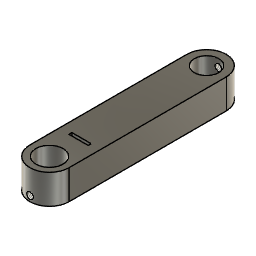
Stirrer Attachment v3 (Autodesk Fusion 360 design; units mm, degrees)
Autodesk Fusion 360 part; units mm, degrees
note: some values were not read from the file. Set by a fixed rule: which face or edge a step refers to.
sketch "Sketch1" plane through (0, 0, 0) normal (0, 0, 1) x (1, 0, 0)
  line L0 (10, -50) -> (-10, -50)
  line L1 (-10, -50) -> (-10, 50)
  line L2 (-10, 50) -> (10, 50)
  line L3 (10, 50) -> (10, -50)
  line L4 (10, -50) -> (-10, 50) construction
  line L5 (-10, -50) -> (10, 50) construction
  circle A0 centre (0, -40) radius 10
  circle A1 centre (0, 40) radius 10
  circle A2 centre (0, -40) radius 6.9
  line L6 (-2.5, -33.1) -> (2.5, -33.1)
  line L7 (0, -33.1) -> (0, -37.8)
  circle A3 centre (0, 40) radius 6.2
  line L8 (-4.7612, -23.8062) -> (5.065, -23.8062)
  line L9 (5.065, -23.8062) -> (5.065, -25.3251)
  line L10 (5.065, -25.3251) -> (-4.7612, -25.3251)
  line L11 (-4.7612, -25.3251) -> (-4.7612, -23.8062)
  dimension "d1" = 100
  dimension "d2" = 20
  dimension "d3" = 13.8
  dimension "d13" = 12.4
  constraint perpendicular L0 L1
  constraint parallel L0 L2
  constraint parallel L1 L3
  constraint horizontal L0
  constraint coincident L4 origin
  constraint coincident L5 origin
  constraint tangent L0 A0
  constraint tangent L1 A0
  constraint tangent L3 A0
  constraint tangent L2 A1
  constraint tangent L1 A1
  constraint tangent L3 A1
  constraint concentric A0 A2
  constraint horizontal L6
  constraint tangent A2 L6
  constraint midpoint L6 L7.start
  constraint perpendicular L6 L7
  constraint concentric A1 A3
  constraint horizontal L8
  constraint vertical L9
  constraint horizontal L10
  constraint vertical L11
  constraint coincident L4 L9.end
  constraint coincident L5 L8.start
  measures "d1" distance of L0.end L1.end
  measures "d2" distance of L1.end L2.end
  measures "d3" diameter of A2
  measures "d13" diameter of A3
extrude "Extrude1" add sketch "Sketch1" along normal blind 15 contours A0 | L1 L3 A0 A1 | A1
ref_plane "WorkPlane1" through (0, -50, 13.2788) normal (0, -1, 0) x (-1, 0, 0)
sketch "Sketch3" plane through (0, -50, 13.2788) normal (0, -1, 0) x (1, 0, 0)
  line L0 (10, -13.2788) -> (-10, -13.2788)
  line L1 (10, -13.2788) -> (10, 1.7212)
  line L2 (10, 1.7212) -> (-10, 1.7212)
  line L3 (-10, 1.7212) -> (-10, -13.2788)
  line L4 (0, -13.2788) -> (0, -10.5788)
  circle A0 centre (0, -10.5788) radius 2
  dimension "d23" = 4
  dimension "d24" = 2.7
  constraint midpoint L0 L4.start
  constraint coincident L4.end A0.centre
  measures "d23" diameter of A0
  measures "d24" distance of L4.start L4.end
extrude "Extrude2" cut sketch "Sketch3" along normal up to surface contours A0 end surface at (6.7055, -38.3733, 10)
thread "Thread4" "ISO Metric profile 4.0 M4x0.7 6H" major diameter 4.1095 minor diameter 3.332 pitch 0.7 angle 60 resizes the face on face at (1.0921, -47.8553, 4.3755)
ref_plane "WorkPlane2" through (0, 50, 7.5255) normal (0, 1, 0) x (1, 0, 0)
sketch "Sketch4" plane through (0, 50, 7.5255) normal (0, 1, 0) x (1, 0, 0)
  line L0 (-10, 7.5255) -> (10, 7.5255)
  line L1 (-10, 7.5255) -> (-10, -7.4745)
  line L2 (-10, -7.4745) -> (10, -7.4745)
  line L3 (10, -7.4745) -> (10, 7.5255)
  line L4 (0, -7.4745) -> (0, 7.5255)
  line L5 (0, -7.4745) -> (0, -3.4745)
  line L6 (0, 7.5255) -> (0, 3.5255)
  circle A0 centre (0, -3.4745) radius 2
  circle A1 centre (0, 3.5255) radius 2
  dimension "d15" = 4
  dimension "d16" = 4
  dimension "d17" = 4
  dimension "d18" = 4
  constraint midpoint L2 L4.start
  constraint midpoint L0 L4.end
  constraint perpendicular L2 L5
  constraint vertical L6
  constraint coincident L5.end A0.centre
  constraint coincident L6.end A1.centre
  measures "d15" distance of L4.start L5.end
  measures "d16" distance of L4.end L6.end
  measures "d17" diameter of A0
  measures "d18" diameter of A1
extrude "Extrude3" cut sketch "Sketch4" along normal up to surface contours L4 L6 A1 | L4 L6 A1 | L4 L5 A0 | L4 L5 A0 end surface at (6.1923, 40.309, 10)
thread "Thread3" "ISO Metric profile 4.0 M4x0.7 6H" major diameter 4.1095 minor diameter 3.332 pitch 0.7 angle 60 resizes the face on face at (0.6977, 48.7045, 9.1256) on face at (0.6977, 48.7045, 2.1256)
ref_plane "WorkPlane3" through (-10, -40, 5.6483) normal (-1, 0, 0) x (0, 1, 0)
sketch "Sketch6" plane through (-10, -40, 5.6483) normal (-1, 0, 0) x (0, 1, 0)
  line L0 (0, -9.3517) -> (0, 5.6483)
  line L1 (0, 5.6483) -> (0, 2.9483)
  circle A0 centre (0, 2.9483) radius 2
  dimension "d27" = 2.7
  dimension "d28" = 4
  constraint coincident L1.end A0.centre
  measures "d27" distance of L0.end L1.end
  measures "d28" diameter of A0
extrude "Extrude4" cut sketch "Sketch6" along normal up to surface end surface at (6.8657, -39.313, 5)
thread "Thread5" "ISO Metric profile 4.0 M4x0.7 6H" major diameter 4.1095 minor diameter 3.332 pitch 0.7 angle 60 resizes the face on face at (-7.9062, -39.2306, 0.8539)
